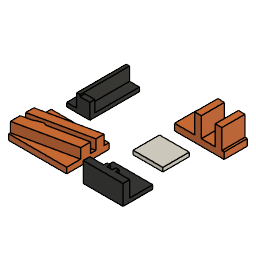
binstack-test-kit (Autodesk Fusion 360 design; units mm, degrees)
part number: 2026-08-18-20-31-15-822
part number: 2026-08-18-20-31-15-985
part number: 2026-08-18-20-31-16-091
part number: 2026-08-18-20-31-16-168
part number: 2026-08-18-20-31-16-285
part number: 2026-08-18-20-31-16-324
Autodesk Fusion 360 part; units mm, degrees
sketch "Sketch1" plane through (0, 0, 0) normal (0, 0, 1) x (1, 0, 0) in component "Купон полоза"
  line L0 (0, 0) -> (35, 0)
  line L1 (35, 0) -> (35, 25.6395)
  line L2 (35, 25.6395) -> (0, 25.6395)
  line L3 (0, 25.6395) -> (0, 0)
extrude "Extrude1" add sketch "Sketch1" along normal blind 3.5 makes body 1 in component "Купон полоза"
sketch "Sketch2" plane through (0, 0, 0) normal (0, 0, 1) x (1, 0, 0) in component "Купон полоза"
  line L0 (0, 1) -> (35, 8.4395)
  line L1 (35, 8.4395) -> (35, 14.4395)
  line L2 (35, 14.4395) -> (0, 7)
  line L3 (0, 7) -> (0, 1)
extrude "Extrude2" add sketch "Sketch2" along normal blind 6 from surface at 3.5 separate body makes body 2 in component "Купон полоза"
sketch "Sketch3" plane through (0, 0, 0) normal (0, 0, 1) x (1, 0, 0) in component "Купон полоза"
  line L0 (0, 10.2) -> (35, 17.6395)
  line L1 (35, 17.6395) -> (35, 22.6395)
  line L2 (35, 22.6395) -> (0, 15.2)
  line L3 (0, 15.2) -> (0, 10.2)
extrude "Extrude3" add sketch "Sketch3" along normal blind 6 from surface at 3.5 separate body makes body 3 in component "Купон полоза"
sketch "Sketch4" plane through (0, 0, 0) normal (0, 0, 1) x (1, 0, 0) in component "Купон полоза"
  line L0 (6, 8.2753) -> (8, 9.2753)
  line L1 (8, 9.2753) -> (11, 10.3381)
  line L2 (11, 10.3381) -> (13, 9.7632)
  line L3 (13, 9.7632) -> (6, 8.2753)
extrude "Extrude4" add sketch "Sketch4" along normal blind 6 from surface at 3.5 separate body makes body 4 in component "Купон полоза"
combine "Combine1" operation add target body 1 tool bodies 2 3 4 in component "Купон полоза"
sketch "Sketch1 (2)" plane through (0, 0, 0) normal (0, 0, 1) x (1, 0, 0) in component "Слайдер с фланцем"
  line L0 (0, 0) -> (14, 0)
  line L1 (14, 0) -> (14, 30)
  line L2 (14, 30) -> (0, 30)
  line L3 (0, 30) -> (0, 0)
extrude "Extrude1'" add sketch "Sketch1 (2)" along normal blind 2.4 separate body makes body 5 in component "Слайдер с фланцем"
sketch "Sketch2 (2)" plane through (0, 0, 0) normal (0, 0, 1) x (1, 0, 0) in component "Слайдер с фланцем"
  line L0 (6, 0) -> (8, 0)
  line L1 (8, 0) -> (8, 30)
  line L2 (8, 30) -> (6, 30)
  line L3 (6, 30) -> (6, 0)
extrude "Extrude2'" add sketch "Sketch2 (2)" along normal blind 8 from surface at 2.4 separate body makes body 6 in component "Слайдер с фланцем"
sketch "Sketch3 (2)" plane through (0, 0, 0) normal (0, 0, 1) x (1, 0, 0) in component "Слайдер с фланцем"
  line L0 (6, 0) -> (14, 0)
  line L1 (14, 0) -> (14, 3)
  line L2 (14, 3) -> (6, 3)
  line L3 (6, 3) -> (6, 0)
extrude "Extrude3'" add sketch "Sketch3 (2)" along normal blind 7 from surface at 2.4 separate body makes body 7 in component "Слайдер с фланцем"
combine "Combine1'" operation add target body 5 tool bodies 6 7 in component "Слайдер с фланцем"
sketch "Sketch1 (3)" plane through (0, 0, 0) normal (0, 0, 1) x (1, 0, 0) in component "Купон паза перегородки"
  line L0 (0, 0) -> (24, 0)
  line L1 (24, 0) -> (24, 18)
  line L2 (24, 18) -> (0, 18)
  line L3 (0, 18) -> (0, 0)
extrude "Extrude1''" add sketch "Sketch1 (3)" along normal blind 2.4 separate body makes body 8 in component "Купон паза перегородки"
sketch "Sketch2 (3)" plane through (0, 0, 0) normal (0, 0, 1) x (1, 0, 0) in component "Купон паза перегородки"
  line L0 (0, 0) -> (24, 0)
  line L1 (24, 0) -> (24, 4)
  line L2 (24, 4) -> (0, 4)
  line L3 (0, 4) -> (0, 0)
extrude "Extrude2''" add sketch "Sketch2 (3)" along normal blind 12 separate body makes body 9 in component "Купон паза перегородки"
sketch "Sketch3 (3)" plane through (0, 0, 0) normal (0, 0, 1) x (1, 0, 0) in component "Купон паза перегородки"
  line L0 (8.4, 4) -> (10.4, 4)
  line L1 (10.4, 4) -> (10.4, 6)
  line L2 (10.4, 6) -> (8.4, 6)
  line L3 (8.4, 6) -> (8.4, 4)
extrude "Extrude3''" add sketch "Sketch3 (3)" along normal blind 9.6 from surface at 2.4 separate body makes body 10 in component "Купон паза перегородки"
sketch "Sketch4 (2)" plane through (0, 0, 0) normal (0, 0, 1) x (1, 0, 0) in component "Купон паза перегородки"
  line L0 (13.6, 4) -> (15.6, 4)
  line L1 (15.6, 4) -> (15.6, 6)
  line L2 (15.6, 6) -> (13.6, 6)
  line L3 (13.6, 6) -> (13.6, 4)
extrude "Extrude4'" add sketch "Sketch4 (2)" along normal blind 9.6 from surface at 2.4 separate body makes body 11 in component "Купон паза перегородки"
combine "Combine1''" operation add target body 8 tool bodies 9 10 11 in component "Купон паза перегородки"
sketch "Sketch1 (4)" plane through (0, 0, 0) normal (0, 0, 1) x (1, 0, 0) in component "Перегородка"
  line L0 (0, 0) -> (18, 0)
  line L1 (18, 0) -> (18, 16)
  line L2 (18, 16) -> (0, 16)
  line L3 (0, 16) -> (0, 0)
extrude "Extrude1'''" add sketch "Sketch1 (4)" along normal blind 2.4 separate body makes body 12 in component "Перегородка"
sketch "Sketch1 (5)" plane through (0, 0, 0) normal (0, 0, 1) x (1, 0, 0) in component "Башмак подставки"
  line L0 (0, 0) -> (30, 0)
  line L1 (30, 0) -> (30, 14)
  line L2 (30, 14) -> (0, 14)
  line L3 (0, 14) -> (0, 0)
extrude "Extrude1''''" add sketch "Sketch1 (5)" along normal blind 4 separate body makes body 13 in component "Башмак подставки"
sketch "Sketch2 (4)" plane through (0, 0, 0) normal (0, 0, 1) x (1, 0, 0) in component "Башмак подставки"
  line L0 (12.2, 0) -> (16.2, 0)
  line L1 (16.2, 0) -> (16.2, 14)
  line L2 (16.2, 14) -> (12.2, 14)
  line L3 (12.2, 14) -> (12.2, 0)
extrude "Extrude2'''" add sketch "Sketch2 (4)" along normal blind 12 from surface at 4 separate body makes body 14 in component "Башмак подставки"
sketch "Sketch3 (4)" plane through (0, 0, 0) normal (0, 0, 1) x (1, 0, 0) in component "Башмак подставки"
  line L0 (24.6, 0) -> (28.6, 0)
  line L1 (28.6, 0) -> (28.6, 14)
  line L2 (28.6, 14) -> (24.6, 14)
  line L3 (24.6, 14) -> (24.6, 0)
extrude "Extrude3'''" add sketch "Sketch3 (4)" along normal blind 12 from surface at 4 separate body makes body 15 in component "Башмак подставки"
combine "Combine1'''" operation add target body 13 tool bodies 14 15 in component "Башмак подставки"
component "Купон полоза" placed x (1, 0, 0) y (0, 1, 0) z (0, 0, 1) at (0, 0, 0)
component "Слайдер с фланцем" placed x (1, 0, 0) y (0, 1, 0) z (0, 0, 1) at (0, 35, 0)
component "Купон паза перегородки" placed x (1, 0, 0) y (0, 1, 0) z (0, 0, 1) at (45, 0, 0)
component "Перегородка" placed x (1, 0, 0) y (0, 1, 0) z (0, 0, 1) at (45, 30, 0)
component "Башмак подставки" placed x (1, 0, 0) y (0, 1, 0) z (0, 0, 1) at (45, 55, 0)
named bodies: "Тело"
